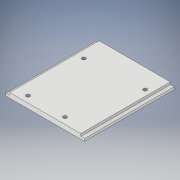
# Autodesk Inventor part: uno-holder
Saved by Autodesk Inventor 2018 (Build 220112000, 112)
## iProperties
Created: 2018-07-29
Part Number: uno-holder
Material: Generic
Document SubType Name: Modeling
Designer: jklei
Density: 1 g/cm^3
Appearance: Default
Author: jklei
Autodesk Inventor part; units mm, degrees
ref_plane "YZ Plane" through (0, 0, 0) normal (1, 0, 0) x (0, 1, 0)
ref_plane "XZ Plane" through (0, 0, 0) normal (0, 1, 0) x (-1, 0, 0)
ref_plane "XY Plane" through (0, 0, 0) normal (0, 0, 1) x (1, 0, 0)
sketch "Sketch1" plane through (0, 0, 0) normal (0, 1, 0) x (-1, 0, 0)
  line L0 (0, 0) -> (-53.5, 0)
  line L1 (-53.5, 0) -> (-53.5, -68.5)
  line L2 (-53.5, -68.5) -> (0, -68.5)
  line L3 (0, -68.5) -> (0, 0)
  dimension "d0" = 53.5
  dimension "d1" = 68.5
  constraints: 8 end point, 2 parallel, 1 horizontal, 1 perpendicular
  measures "d0" distance of L2.end L1.end
  measures "d1" distance of L1.end L0.end
extrude "Extrusion1" add sketch "Sketch1" along normal blind 4
sketch "Sketch2" plane through (0, 4, 0) normal (0, 1, 0) x (1, 0, 0)
  circle A0 centre (51, 55.0126) radius 1.5
  line L0 (53.5, 68.5) -> (0, 68.5) projected
  line L1 (53.5, 0) -> (53.5, 68.5) projected
  circle A1 centre (4, 52) radius 1.5
  line L2 (0, 68.5) -> (0, 0) projected
  circle A2 centre (37.7012, 3) radius 1.5
  line L3 (0, 0) -> (53.5, 0) projected
  circle A3 centre (7.493, 3) radius 1.5
  dimension "d4" = 3
  dimension "d5" = 13.4874
  dimension "d6" = 2.5
  dimension "d7" = 3
  dimension "d8" = 16.5
  dimension "d9" = 4
  dimension "d10" = 3
  dimension "d11" = 15.7988
  dimension "d12" = 3
  dimension "d13" = 3
  dimension "d14" = 3
  dimension "d15" = 7.493
  constraints: 4 centre point
  measures "d4" diameter of A0
  measures "d5" distance from line of A0.centre L0
  measures "d6" distance from line of L1 A0.centre
  measures "d7" diameter of A1
  measures "d8" distance from line of L0 A1.centre
  measures "d9" distance from line of L2 A1.centre
  measures "d10" diameter of A2
  measures "d11" distance from line of L1 A2.centre
  measures "d12" distance from line of L3 A2.centre
  measures "d13" diameter of A3
  measures "d14" distance from line of L3 A3.centre
  measures "d15" distance from line of L2 A3.centre
extrude "Extrusion2" cut sketch "Sketch2" against normal blind 12 contours A0 | A1 | A2 | A3
sketch "Sketch3" plane through (0, 4, 0) normal (0, 1, 0) x (1, 0, 0)
  line L0 (0, 0) -> (53.5, 0) projected
  line L1 (53.5, 0) -> (53.5, 68.5) projected
  line L2 (53.5, 68.5) -> (0, 68.5) projected
  line L3 (0, 68.5) -> (0, 0) projected
  line L4 (-2.25, -2.25) -> (55.75, -2.25)
  line L5 (55.75, -2.25) -> (55.75, 70.75)
  line L6 (55.75, 70.75) -> (-2.25, 70.75)
  line L7 (-2.25, 70.75) -> (-2.25, -2.25)
  dimension "d18" = 2.25
  constraints: 8 end point, 3 other
  measures "d18" distance between parallel lines of L3 L7
extrude "Extrusion3" add sketch "Sketch3" against normal blind 4
sketch "Sketch6" plane through (55.75, 4, 2.25) normal (1, 0, 0) x (0, 0, -1)
  line L0 (0, 0) -> (73, 0) projected
  line L1 (73, -4) -> (0, -4) projected
  line L2 (0, 0) -> (73, 0) projected
  line L3 (0, 0) -> (0, -4) projected
  line L4 (73, -4) -> (0, -4) projected
  line L5 (73, 0) -> (73, -4) projected
  line L6 (73, 0) -> (73, -4) projected
  line L7 (0, -4) -> (73, -4)
  line L8 (73, -4) -> (73, -2)
  line L9 (73, -2) -> (0, -2)
  line L10 (0, -2) -> (0, -4)
  point P0 (2.25, -4)
  dimension "d33" = 2
  constraints: 8 end point, 2 parallel, 1 horizontal, 1 midpoint, 1 perpendicular
  measures "d33" distance of L8.end L7.end
extrude "Extrusion6" add sketch "Sketch6" along normal blind 3 contours L9 L5 L1 L3
sketch "Sketch7" plane through (-2.25, 4, -70.75) normal (-1, 0, 0) x (0, 0, 1)
  line L0 (73, -4) -> (0, -4) projected
  line L1 (0, -4) -> (0, -2) projected
  line L2 (0, -2) -> (73, -2) projected
  line L3 (73, -2) -> (73, -4) projected
  point P0 (70.75, -4)
extrude "Extrusion7" add sketch "Sketch7" along normal blind 3
body "Solid1"
